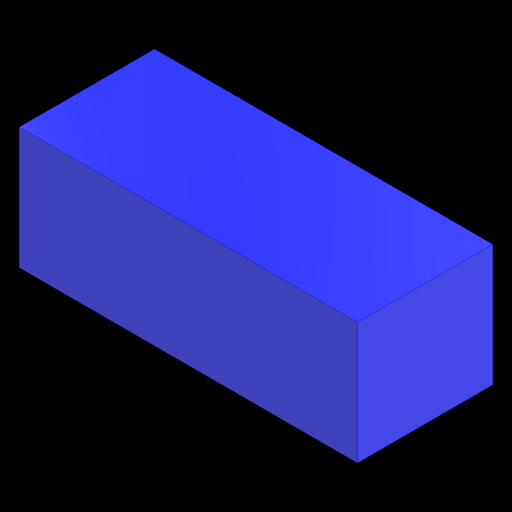
# Autodesk Inventor part: BatteryMockup
Saved by Autodesk Inventor 2023 (Build 270158000, 158)
## iProperties
Created: 2021-02-15
Part Number: BatteryMockup
Material: Generic
Document SubType Name: Modeling
Designer: Esketitttttt
Density: 1.37727 g/cm^3
Appearance: Blue - Wall Paint - Glossy
Mass: 26 g
Surface Area: 46.658 cm^2
Volume: 18.8779 cm^3
Author: Esketitttttt
Autodesk Inventor part; units mm, degrees
ref_plane "YZ Plane" through (0, 0, 0) normal (1, 0, 0) x (0, 1, 0)
ref_plane "XZ Plane" through (0, 0, 0) normal (0, 1, 0) x (-1, 0, 0)
ref_plane "XY Plane" through (0, 0, 0) normal (0, 0, 1) x (1, 0, 0)
sketch "Sketch1" plane through (0, 0, 0) normal (0, 1, 0) x (-1, 0, 0)
  line L0 (0, 0) -> (50.8, 0)
  line L1 (50.8, 0) -> (50.8, -20.32)
  line L2 (50.8, -20.32) -> (0, -20.32)
  line L3 (0, -20.32) -> (0, 0)
  dimension "d0" = 50.8
  dimension "d1" = 20.32
  constraints: 8 end point, 2 parallel, 1 horizontal, 1 perpendicular
  measures "d0" distance of L1.end L2.end
  measures "d1" distance of L0.end L1.end
extrude "Extrusion1" add sketch "Sketch1" along normal blind 18.288
body "Solid1"
